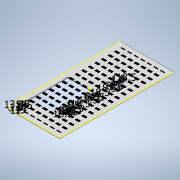
# Autodesk Inventor part: Backboard
Saved by Autodesk Inventor 2021 (Build 250183000, 183)
## iProperties
Created: 2020-06-05
Part Number: Backboard
Material: Generic
Document SubType Name: Modeling
Designer: ameli
Density: 1 g/cm^3
Appearance: Default
Author: ameli
Autodesk Inventor part; units mm, degrees
ref_plane "YZ Plane" through (0, 0, 0) normal (1, 0, 0) x (0, 1, 0)
ref_plane "XZ Plane" through (0, 0, 0) normal (0, 1, 0) x (-1, 0, 0)
ref_plane "XY Plane" through (0, 0, 0) normal (0, 0, 1) x (1, 0, 0)
sketch "Sketch1" plane through (0, 0, 0) normal (0, 1, 0) x (-1, 0, 0)
  line L0 (62, 129.5) -> (-60.5, 129.5)
  line L1 (-60.5, 129.5) -> (-60.5, -131.5)
  line L2 (-60.5, -131.5) -> (62, -131.5)
  line L3 (62, -131.5) -> (62, 129.5)
  point P0 (0, 0)
  dimension "d0" = 122.5
  dimension "d1" = 261
  dimension "d2" = 62
  dimension "d3" = 129.5
  constraints: 8 end point, 2 parallel, 1 horizontal, 1 perpendicular
  measures "d0" distance of L0.start L0.end
  measures "d1" distance of L2.end L0.start
  measures "d2" distance from line of point (0, 0) L3
  measures "d3" distance from line of point (0, 0) L0
extrude "Extrusion1" add sketch "Sketch1" along normal blind 2
sketch "Sketch6" plane through (0, 2, 0) normal (0, 1, 0) x (1, 0, 0)
  line L0 (-51, -88.5) -> (6, -88.5)
  line L1 (6, -88.5) -> (6, 0.5)
  line L2 (6, 0.5) -> (-51, 0.5)
  line L3 (-51, 0.5) -> (-51, -88.5)
  line L4 (-62, 131.5) -> (-62, -129.5) projected
  line L5 (-62, -129.5) -> (60.5, -129.5) projected
  point P0 (0, 0)
  dimension "d22" = 89
  dimension "d23" = 57
  dimension "d24" = 11
  dimension "d25" = 41
  constraints: 8 end point, 2 parallel, 1 horizontal, 1 perpendicular
  measures "d22" distance of L2.end L0.start
  measures "d23" distance of L0.start L0.end
  measures "d24" distance between parallel lines of L4 L3
  measures "d25" distance between parallel lines of L5 L0
extrude "Extrusion2" cut sketch "Sketch6" against normal blind 10
sketch "Sketch10" plane through (0, 2, 0) normal (0, 1, 0) x (1, 0, 0)
  line L0 (-48.25, -118.5) -> (-39.75, -118.5)
  line L1 (-39.75, -118.5) -> (-39.75, -117)
  line L2 (-39.75, -117) -> (-48.25, -117)
  line L3 (-48.25, -117) -> (-48.25, -118.5)
  line L4 (-48.25, -106) -> (-39.75, -106)
  line L5 (-39.75, -106) -> (-39.75, -104.5)
  line L6 (-39.75, -104.5) -> (-48.25, -104.5)
  line L7 (-48.25, -104.5) -> (-48.25, -106)
  line L8 (-62, 131.5) -> (-62, -129.5) projected
  line L9 (-62, -129.5) -> (60.5, -129.5) projected
  line L10 (-48.25, -103.5) -> (-39.75, -103.5)
  line L11 (-39.75, -103.5) -> (-39.75, -102)
  line L12 (-39.75, -102) -> (-48.25, -102)
  line L13 (-48.25, -102) -> (-48.25, -103.5)
  line L14 (-48.25, -91) -> (-39.75, -91)
  line L15 (-39.75, -91) -> (-39.75, -89.5)
  line L16 (-39.75, -89.5) -> (-48.25, -89.5)
  line L17 (-48.25, -89.5) -> (-48.25, -91)
  line L18 (-48.25, -88.5) -> (-39.75, -88.5)
  line L19 (-39.75, -88.5) -> (-39.75, -87)
  line L20 (-39.75, -87) -> (-48.25, -87)
  line L21 (-48.25, -87) -> (-48.25, -88.5)
  line L22 (-48.25, -76) -> (-39.75, -76)
  line L23 (-39.75, -76) -> (-39.75, -74.5)
  line L24 (-39.75, -74.5) -> (-48.25, -74.5)
  line L25 (-48.25, -74.5) -> (-48.25, -76)
  line L26 (-48.25, -73.5) -> (-39.75, -73.5)
  line L27 (-39.75, -73.5) -> (-39.75, -72)
  line L28 (-39.75, -72) -> (-48.25, -72)
  line L29 (-48.25, -72) -> (-48.25, -73.5)
  line L30 (-48.25, -61) -> (-39.75, -61)
  line L31 (-39.75, -61) -> (-39.75, -59.5)
  line L32 (-39.75, -59.5) -> (-48.25, -59.5)
  line L33 (-48.25, -59.5) -> (-48.25, -61)
  line L34 (-48.25, -58.5) -> (-39.75, -58.5)
  line L35 (-39.75, -58.5) -> (-39.75, -57)
  line L36 (-39.75, -57) -> (-48.25, -57)
  line L37 (-48.25, -57) -> (-48.25, -58.5)
  line L38 (-48.25, -46) -> (-39.75, -46)
  line L39 (-39.75, -46) -> (-39.75, -44.5)
  line L40 (-39.75, -44.5) -> (-48.25, -44.5)
  line L41 (-48.25, -44.5) -> (-48.25, -46)
  line L42 (-48.25, -43.5) -> (-39.75, -43.5)
  line L43 (-39.75, -43.5) -> (-39.75, -42)
  line L44 (-39.75, -42) -> (-48.25, -42)
  line L45 (-48.25, -42) -> (-48.25, -43.5)
  line L46 (-48.25, -31) -> (-39.75, -31)
  line L47 (-39.75, -31) -> (-39.75, -29.5)
  line L48 (-39.75, -29.5) -> (-48.25, -29.5)
  line L49 (-48.25, -29.5) -> (-48.25, -31)
  line L50 (-48.25, -28.5) -> (-39.75, -28.5)
  line L51 (-39.75, -28.5) -> (-39.75, -27)
  line L52 (-39.75, -27) -> (-48.25, -27)
  line L53 (-48.25, -27) -> (-48.25, -28.5)
  line L54 (-48.25, -16) -> (-39.75, -16)
  line L55 (-39.75, -16) -> (-39.75, -14.5)
  line L56 (-39.75, -14.5) -> (-48.25, -14.5)
  line L57 (-48.25, -14.5) -> (-48.25, -16)
  line L58 (-48.25, -13.5) -> (-39.75, -13.5)
  line L59 (-39.75, -13.5) -> (-39.75, -12)
  line L60 (-39.75, -12) -> (-48.25, -12)
  line L61 (-48.25, -12) -> (-48.25, -13.5)
  line L62 (-48.25, -1) -> (-39.75, -1)
  line L63 (-39.75, -1) -> (-39.75, 0.5)
  line L64 (-39.75, 0.5) -> (-48.25, 0.5)
  line L65 (-48.25, 0.5) -> (-48.25, -1)
  line L66 (-48.25, 1.5) -> (-39.75, 1.5)
  line L67 (-39.75, 1.5) -> (-39.75, 3)
  line L68 (-39.75, 3) -> (-48.25, 3)
  line L69 (-48.25, 3) -> (-48.25, 1.5)
  line L70 (-48.25, 14) -> (-39.75, 14)
  line L71 (-39.75, 14) -> (-39.75, 15.5)
  line L72 (-39.75, 15.5) -> (-48.25, 15.5)
  line L73 (-48.25, 15.5) -> (-48.25, 14)
  line L74 (-48.25, 16.5) -> (-39.75, 16.5)
  line L75 (-39.75, 16.5) -> (-39.75, 18)
  line L76 (-39.75, 18) -> (-48.25, 18)
  line L77 (-48.25, 18) -> (-48.25, 16.5)
  line L78 (-48.25, 29) -> (-39.75, 29)
  line L79 (-39.75, 29) -> (-39.75, 30.5)
  line L80 (-39.75, 30.5) -> (-48.25, 30.5)
  line L81 (-48.25, 30.5) -> (-48.25, 29)
  line L82 (-48.25, 31.5) -> (-39.75, 31.5)
  line L83 (-39.75, 31.5) -> (-39.75, 33)
  line L84 (-39.75, 33) -> (-48.25, 33)
  line L85 (-48.25, 33) -> (-48.25, 31.5)
  line L86 (-48.25, 44) -> (-39.75, 44)
  line L87 (-39.75, 44) -> (-39.75, 45.5)
  line L88 (-39.75, 45.5) -> (-48.25, 45.5)
  line L89 (-48.25, 45.5) -> (-48.25, 44)
  line L90 (-48.25, 46.5) -> (-39.75, 46.5)
  line L91 (-39.75, 46.5) -> (-39.75, 48)
  line L92 (-39.75, 48) -> (-48.25, 48)
  line L93 (-48.25, 48) -> (-48.25, 46.5)
  line L94 (-48.25, 59) -> (-39.75, 59)
  line L95 (-39.75, 59) -> (-39.75, 60.5)
  line L96 (-39.75, 60.5) -> (-48.25, 60.5)
  line L97 (-48.25, 60.5) -> (-48.25, 59)
  line L98 (-48.25, 61.5) -> (-39.75, 61.5)
  line L99 (-39.75, 61.5) -> (-39.75, 63)
  line L100 (-39.75, 63) -> (-48.25, 63)
  line L101 (-48.25, 63) -> (-48.25, 61.5)
  line L102 (-48.25, 74) -> (-39.75, 74)
  line L103 (-39.75, 74) -> (-39.75, 75.5)
  line L104 (-39.75, 75.5) -> (-48.25, 75.5)
  line L105 (-48.25, 75.5) -> (-48.25, 74)
  line L106 (-48.25, 76.5) -> (-39.75, 76.5)
  line L107 (-39.75, 76.5) -> (-39.75, 78)
  line L108 (-39.75, 78) -> (-48.25, 78)
  line L109 (-48.25, 78) -> (-48.25, 76.5)
  line L110 (-48.25, 89) -> (-39.75, 89)
  line L111 (-39.75, 89) -> (-39.75, 90.5)
  line L112 (-39.75, 90.5) -> (-48.25, 90.5)
  line L113 (-48.25, 90.5) -> (-48.25, 89)
  line L114 (-48.25, 91.5) -> (-39.75, 91.5)
  line L115 (-39.75, 91.5) -> (-39.75, 93)
  line L116 (-39.75, 93) -> (-48.25, 93)
  line L117 (-48.25, 93) -> (-48.25, 91.5)
  line L118 (-48.25, 104) -> (-39.75, 104)
  line L119 (-39.75, 104) -> (-39.75, 105.5)
  line L120 (-39.75, 105.5) -> (-48.25, 105.5)
  line L121 (-48.25, 105.5) -> (-48.25, 104)
  line L122 (-48.25, 106.5) -> (-39.75, 106.5)
  line L123 (-39.75, 106.5) -> (-39.75, 108)
  line L124 (-39.75, 108) -> (-48.25, 108)
  line L125 (-48.25, 108) -> (-48.25, 106.5)
  line L126 (-48.25, 119) -> (-39.75, 119)
  line L127 (-39.75, 119) -> (-39.75, 120.5)
  line L128 (-39.75, 120.5) -> (-48.25, 120.5)
  line L129 (-48.25, 120.5) -> (-48.25, 119)
  line L130 (-33.25, -118.5) -> (-24.75, -118.5)
  line L131 (-24.75, -118.5) -> (-24.75, -117)
  line L132 (-24.75, -117) -> (-33.25, -117)
  line L133 (-33.25, -117) -> (-33.25, -118.5)
  line L134 (-33.25, -106) -> (-24.75, -106)
  line L135 (-24.75, -106) -> (-24.75, -104.5)
  line L136 (-24.75, -104.5) -> (-33.25, -104.5)
  line L137 (-33.25, -104.5) -> (-33.25, -106)
  line L138 (-33.25, -103.5) -> (-24.75, -103.5)
  line L139 (-24.75, -103.5) -> (-24.75, -102)
  line L140 (-24.75, -102) -> (-33.25, -102)
  line L141 (-33.25, -102) -> (-33.25, -103.5)
  line L142 (-33.25, -91) -> (-24.75, -91)
  line L143 (-24.75, -91) -> (-24.75, -89.5)
  line L144 (-24.75, -89.5) -> (-33.25, -89.5)
  line L145 (-33.25, -89.5) -> (-33.25, -91)
  line L146 (-33.25, -88.5) -> (-24.75, -88.5)
  line L147 (-24.75, -88.5) -> (-24.75, -87)
  line L148 (-24.75, -87) -> (-33.25, -87)
  line L149 (-33.25, -87) -> (-33.25, -88.5)
  line L150 (-33.25, -76) -> (-24.75, -76)
  line L151 (-24.75, -76) -> (-24.75, -74.5)
  line L152 (-24.75, -74.5) -> (-33.25, -74.5)
  line L153 (-33.25, -74.5) -> (-33.25, -76)
  line L154 (-33.25, -73.5) -> (-24.75, -73.5)
  line L155 (-24.75, -73.5) -> (-24.75, -72)
  line L156 (-24.75, -72) -> (-33.25, -72)
  line L157 (-33.25, -72) -> (-33.25, -73.5)
  line L158 (-33.25, -61) -> (-24.75, -61)
  line L159 (-24.75, -61) -> (-24.75, -59.5)
  line L160 (-24.75, -59.5) -> (-33.25, -59.5)
  line L161 (-33.25, -59.5) -> (-33.25, -61)
  line L162 (-33.25, -58.5) -> (-24.75, -58.5)
  line L163 (-24.75, -58.5) -> (-24.75, -57)
  line L164 (-24.75, -57) -> (-33.25, -57)
  line L165 (-33.25, -57) -> (-33.25, -58.5)
  line L166 (-33.25, -46) -> (-24.75, -46)
  line L167 (-24.75, -46) -> (-24.75, -44.5)
  line L168 (-24.75, -44.5) -> (-33.25, -44.5)
  line L169 (-33.25, -44.5) -> (-33.25, -46)
  line L170 (-33.25, -43.5) -> (-24.75, -43.5)
  line L171 (-24.75, -43.5) -> (-24.75, -42)
  line L172 (-24.75, -42) -> (-33.25, -42)
  line L173 (-33.25, -42) -> (-33.25, -43.5)
  line L174 (-33.25, -31) -> (-24.75, -31)
  line L175 (-24.75, -31) -> (-24.75, -29.5)
  line L176 (-24.75, -29.5) -> (-33.25, -29.5)
  line L177 (-33.25, -29.5) -> (-33.25, -31)
  line L178 (-33.25, -28.5) -> (-24.75, -28.5)
  line L179 (-24.75, -28.5) -> (-24.75, -27)
  line L180 (-24.75, -27) -> (-33.25, -27)
  line L181 (-33.25, -27) -> (-33.25, -28.5)
  line L182 (-33.25, -16) -> (-24.75, -16)
  line L183 (-24.75, -16) -> (-24.75, -14.5)
  line L184 (-24.75, -14.5) -> (-33.25, -14.5)
  line L185 (-33.25, -14.5) -> (-33.25, -16)
  line L186 (-33.25, -13.5) -> (-24.75, -13.5)
  line L187 (-24.75, -13.5) -> (-24.75, -12)
  line L188 (-24.75, -12) -> (-33.25, -12)
  line L189 (-33.25, -12) -> (-33.25, -13.5)
  line L190 (-33.25, -1) -> (-24.75, -1)
  line L191 (-24.75, -1) -> (-24.75, 0.5)
  line L192 (-24.75, 0.5) -> (-33.25, 0.5)
  line L193 (-33.25, 0.5) -> (-33.25, -1)
  line L194 (-33.25, 1.5) -> (-24.75, 1.5)
  line L195 (-24.75, 1.5) -> (-24.75, 3)
  line L196 (-24.75, 3) -> (-33.25, 3)
  line L197 (-33.25, 3) -> (-33.25, 1.5)
  line L198 (-33.25, 14) -> (-24.75, 14)
  line L199 (-24.75, 14) -> (-24.75, 15.5)
  line L200 (-24.75, 15.5) -> (-33.25, 15.5)
  line L201 (-33.25, 15.5) -> (-33.25, 14)
  line L202 (-33.25, 16.5) -> (-24.75, 16.5)
  line L203 (-24.75, 16.5) -> (-24.75, 18)
  line L204 (-24.75, 18) -> (-33.25, 18)
  line L205 (-33.25, 18) -> (-33.25, 16.5)
  line L206 (-33.25, 29) -> (-24.75, 29)
  line L207 (-24.75, 29) -> (-24.75, 30.5)
  line L208 (-24.75, 30.5) -> (-33.25, 30.5)
  line L209 (-33.25, 30.5) -> (-33.25, 29)
  line L210 (-33.25, 31.5) -> (-24.75, 31.5)
  line L211 (-24.75, 31.5) -> (-24.75, 33)
  line L212 (-24.75, 33) -> (-33.25, 33)
  line L213 (-33.25, 33) -> (-33.25, 31.5)
  line L214 (-33.25, 44) -> (-24.75, 44)
  line L215 (-24.75, 44) -> (-24.75, 45.5)
  line L216 (-24.75, 45.5) -> (-33.25, 45.5)
  line L217 (-33.25, 45.5) -> (-33.25, 44)
  line L218 (-33.25, 46.5) -> (-24.75, 46.5)
  line L219 (-24.75, 46.5) -> (-24.75, 48)
  line L220 (-24.75, 48) -> (-33.25, 48)
  line L221 (-33.25, 48) -> (-33.25, 46.5)
  line L222 (-33.25, 59) -> (-24.75, 59)
  line L223 (-24.75, 59) -> (-24.75, 60.5)
  line L224 (-24.75, 60.5) -> (-33.25, 60.5)
  line L225 (-33.25, 60.5) -> (-33.25, 59)
  line L226 (-33.25, 61.5) -> (-24.75, 61.5)
  line L227 (-24.75, 61.5) -> (-24.75, 63)
  line L228 (-24.75, 63) -> (-33.25, 63)
  line L229 (-33.25, 63) -> (-33.25, 61.5)
  line L230 (-33.25, 74) -> (-24.75, 74)
  line L231 (-24.75, 74) -> (-24.75, 75.5)
  line L232 (-24.75, 75.5) -> (-33.25, 75.5)
  line L233 (-33.25, 75.5) -> (-33.25, 74)
  line L234 (-33.25, 76.5) -> (-24.75, 76.5)
  line L235 (-24.75, 76.5) -> (-24.75, 78)
  line L236 (-24.75, 78) -> (-33.25, 78)
  line L237 (-33.25, 78) -> (-33.25, 76.5)
  line L238 (-33.25, 89) -> (-24.75, 89)
  line L239 (-24.75, 89) -> (-24.75, 90.5)
  line L240 (-24.75, 90.5) -> (-33.25, 90.5)
  line L241 (-33.25, 90.5) -> (-33.25, 89)
  line L242 (-33.25, 91.5) -> (-24.75, 91.5)
  line L243 (-24.75, 91.5) -> (-24.75, 93)
  line L244 (-24.75, 93) -> (-33.25, 93)
  line L245 (-33.25, 93) -> (-33.25, 91.5)
  line L246 (-33.25, 104) -> (-24.75, 104)
  line L247 (-24.75, 104) -> (-24.75, 105.5)
  line L248 (-24.75, 105.5) -> (-33.25, 105.5)
  line L249 (-33.25, 105.5) -> (-33.25, 104)
  line L250 (-33.25, 106.5) -> (-24.75, 106.5)
  line L251 (-24.75, 106.5) -> (-24.75, 108)
  line L252 (-24.75, 108) -> (-33.25, 108)
  line L253 (-33.25, 108) -> (-33.25, 106.5)
  line L254 (-33.25, 119) -> (-24.75, 119)
  line L255 (-24.75, 119) -> (-24.75, 120.5)
  line L256 (-24.75, 120.5) -> (-33.25, 120.5)
  line L257 (-33.25, 120.5) -> (-33.25, 119)
  line L258 (-18.25, -118.5) -> (-9.75, -118.5)
  line L259 (-9.75, -118.5) -> (-9.75, -117)
  line L260 (-9.75, -117) -> (-18.25, -117)
  line L261 (-18.25, -117) -> (-18.25, -118.5)
  line L262 (-18.25, -106) -> (-9.75, -106)
  line L263 (-9.75, -106) -> (-9.75, -104.5)
  line L264 (-9.75, -104.5) -> (-18.25, -104.5)
  line L265 (-18.25, -104.5) -> (-18.25, -106)
  line L266 (-18.25, -103.5) -> (-9.75, -103.5)
  line L267 (-9.75, -103.5) -> (-9.75, -102)
  line L268 (-9.75, -102) -> (-18.25, -102)
  line L269 (-18.25, -102) -> (-18.25, -103.5)
  line L270 (-18.25, -91) -> (-9.75, -91)
  line L271 (-9.75, -91) -> (-9.75, -89.5)
  line L272 (-9.75, -89.5) -> (-18.25, -89.5)
  line L273 (-18.25, -89.5) -> (-18.25, -91)
  line L274 (-18.25, -88.5) -> (-9.75, -88.5)
  line L275 (-9.75, -88.5) -> (-9.75, -87)
  line L276 (-9.75, -87) -> (-18.25, -87)
  line L277 (-18.25, -87) -> (-18.25, -88.5)
  line L278 (-18.25, -76) -> (-9.75, -76)
  line L279 (-9.75, -76) -> (-9.75, -74.5)
  line L280 (-9.75, -74.5) -> (-18.25, -74.5)
  line L281 (-18.25, -74.5) -> (-18.25, -76)
  line L282 (-18.25, -73.5) -> (-9.75, -73.5)
  line L283 (-9.75, -73.5) -> (-9.75, -72)
  line L284 (-9.75, -72) -> (-18.25, -72)
  line L285 (-18.25, -72) -> (-18.25, -73.5)
  line L286 (-18.25, -61) -> (-9.75, -61)
  line L287 (-9.75, -61) -> (-9.75, -59.5)
  line L288 (-9.75, -59.5) -> (-18.25, -59.5)
  line L289 (-18.25, -59.5) -> (-18.25, -61)
  line L290 (-18.25, -58.5) -> (-9.75, -58.5)
  line L291 (-9.75, -58.5) -> (-9.75, -57)
  line L292 (-9.75, -57) -> (-18.25, -57)
  line L293 (-18.25, -57) -> (-18.25, -58.5)
  line L294 (-18.25, -46) -> (-9.75, -46)
  line L295 (-9.75, -46) -> (-9.75, -44.5)
  line L296 (-9.75, -44.5) -> (-18.25, -44.5)
  line L297 (-18.25, -44.5) -> (-18.25, -46)
  line L298 (-18.25, -43.5) -> (-9.75, -43.5)
  line L299 (-9.75, -43.5) -> (-9.75, -42)
  line L300 (-9.75, -42) -> (-18.25, -42)
  line L301 (-18.25, -42) -> (-18.25, -43.5)
  line L302 (-18.25, -31) -> (-9.75, -31)
  line L303 (-9.75, -31) -> (-9.75, -29.5)
  line L304 (-9.75, -29.5) -> (-18.25, -29.5)
  line L305 (-18.25, -29.5) -> (-18.25, -31)
  line L306 (-18.25, -28.5) -> (-9.75, -28.5)
  line L307 (-9.75, -28.5) -> (-9.75, -27)
  line L308 (-9.75, -27) -> (-18.25, -27)
  line L309 (-18.25, -27) -> (-18.25, -28.5)
  line L310 (-18.25, -16) -> (-9.75, -16)
  line L311 (-9.75, -16) -> (-9.75, -14.5)
  line L312 (-9.75, -14.5) -> (-18.25, -14.5)
  line L313 (-18.25, -14.5) -> (-18.25, -16)
  line L314 (-18.25, -13.5) -> (-9.75, -13.5)
  line L315 (-9.75, -13.5) -> (-9.75, -12)
  line L316 (-9.75, -12) -> (-18.25, -12)
  line L317 (-18.25, -12) -> (-18.25, -13.5)
  line L318 (-18.25, -1) -> (-9.75, -1)
  line L319 (-9.75, -1) -> (-9.75, 0.5)
  line L320 (-9.75, 0.5) -> (-18.25, 0.5)
  line L321 (-18.25, 0.5) -> (-18.25, -1)
  line L322 (-18.25, 1.5) -> (-9.75, 1.5)
  line L323 (-9.75, 1.5) -> (-9.75, 3)
  line L324 (-9.75, 3) -> (-18.25, 3)
  line L325 (-18.25, 3) -> (-18.25, 1.5)
  line L326 (-18.25, 14) -> (-9.75, 14)
  line L327 (-9.75, 14) -> (-9.75, 15.5)
  line L328 (-9.75, 15.5) -> (-18.25, 15.5)
  line L329 (-18.25, 15.5) -> (-18.25, 14)
  line L330 (-18.25, 16.5) -> (-9.75, 16.5)
  line L331 (-9.75, 16.5) -> (-9.75, 18)
  line L332 (-9.75, 18) -> (-18.25, 18)
  line L333 (-18.25, 18) -> (-18.25, 16.5)
  line L334 (-18.25, 29) -> (-9.75, 29)
  line L335 (-9.75, 29) -> (-9.75, 30.5)
  line L336 (-9.75, 30.5) -> (-18.25, 30.5)
  line L337 (-18.25, 30.5) -> (-18.25, 29)
  line L338 (-18.25, 31.5) -> (-9.75, 31.5)
  line L339 (-9.75, 31.5) -> (-9.75, 33)
  line L340 (-9.75, 33) -> (-18.25, 33)
  line L341 (-18.25, 33) -> (-18.25, 31.5)
  line L342 (-18.25, 44) -> (-9.75, 44)
  line L343 (-9.75, 44) -> (-9.75, 45.5)
  line L344 (-9.75, 45.5) -> (-18.25, 45.5)
  line L345 (-18.25, 45.5) -> (-18.25, 44)
  line L346 (-18.25, 46.5) -> (-9.75, 46.5)
  line L347 (-9.75, 46.5) -> (-9.75, 48)
  line L348 (-9.75, 48) -> (-18.25, 48)
  line L349 (-18.25, 48) -> (-18.25, 46.5)
  line L350 (-18.25, 59) -> (-9.75, 59)
  line L351 (-9.75, 59) -> (-9.75, 60.5)
  line L352 (-9.75, 60.5) -> (-18.25, 60.5)
  line L353 (-18.25, 60.5) -> (-18.25, 59)
  line L354 (-18.25, 61.5) -> (-9.75, 61.5)
  line L355 (-9.75, 61.5) -> (-9.75, 63)
  line L356 (-9.75, 63) -> (-18.25, 63)
  line L357 (-18.25, 63) -> (-18.25, 61.5)
  line L358 (-18.25, 74) -> (-9.75, 74)
  line L359 (-9.75, 74) -> (-9.75, 75.5)
  line L360 (-9.75, 75.5) -> (-18.25, 75.5)
  line L361 (-18.25, 75.5) -> (-18.25, 74)
  line L362 (-18.25, 76.5) -> (-9.75, 76.5)
  line L363 (-9.75, 76.5) -> (-9.75, 78)
  line L364 (-9.75, 78) -> (-18.25, 78)
  line L365 (-18.25, 78) -> (-18.25, 76.5)
  line L366 (-18.25, 89) -> (-9.75, 89)
  line L367 (-9.75, 89) -> (-9.75, 90.5)
  line L368 (-9.75, 90.5) -> (-18.25, 90.5)
  line L369 (-18.25, 90.5) -> (-18.25, 89)
  line L370 (-18.25, 91.5) -> (-9.75, 91.5)
  line L371 (-9.75, 91.5) -> (-9.75, 93)
  line L372 (-9.75, 93) -> (-18.25, 93)
  line L373 (-18.25, 93) -> (-18.25, 91.5)
  line L374 (-18.25, 104) -> (-9.75, 104)
  line L375 (-9.75, 104) -> (-9.75, 105.5)
  line L376 (-9.75, 105.5) -> (-18.25, 105.5)
  line L377 (-18.25, 105.5) -> (-18.25, 104)
  line L378 (-18.25, 106.5) -> (-9.75, 106.5)
  line L379 (-9.75, 106.5) -> (-9.75, 108)
  line L380 (-9.75, 108) -> (-18.25, 108)
  line L381 (-18.25, 108) -> (-18.25, 106.5)
  line L382 (-18.25, 119) -> (-9.75, 119)
  line L383 (-9.75, 119) -> (-9.75, 120.5)
  line L384 (-9.75, 120.5) -> (-18.25, 120.5)
  line L385 (-18.25, 120.5) -> (-18.25, 119)
  line L386 (-3.25, -118.5) -> (5.25, -118.5)
  line L387 (5.25, -118.5) -> (5.25, -117)
  line L388 (5.25, -117) -> (-3.25, -117)
  line L389 (-3.25, -117) -> (-3.25, -118.5)
  line L390 (-3.25, -106) -> (5.25, -106)
  line L391 (5.25, -106) -> (5.25, -104.5)
  line L392 (5.25, -104.5) -> (-3.25, -104.5)
  line L393 (-3.25, -104.5) -> (-3.25, -106)
  line L394 (-3.25, -103.5) -> (5.25, -103.5)
  line L395 (5.25, -103.5) -> (5.25, -102)
  line L396 (5.25, -102) -> (-3.25, -102)
  line L397 (-3.25, -102) -> (-3.25, -103.5)
  line L398 (-3.25, -91) -> (5.25, -91)
  line L399 (5.25, -91) -> (5.25, -89.5)
  line L400 (5.25, -89.5) -> (-3.25, -89.5)
  line L401 (-3.25, -89.5) -> (-3.25, -91)
  line L402 (-3.25, -88.5) -> (5.25, -88.5)
  line L403 (5.25, -88.5) -> (5.25, -87)
  line L404 (5.25, -87) -> (-3.25, -87)
  line L405 (-3.25, -87) -> (-3.25, -88.5)
  line L406 (-3.25, -76) -> (5.25, -76)
  line L407 (5.25, -76) -> (5.25, -74.5)
  line L408 (5.25, -74.5) -> (-3.25, -74.5)
  line L409 (-3.25, -74.5) -> (-3.25, -76)
  line L410 (-3.25, -73.5) -> (5.25, -73.5)
  line L411 (5.25, -73.5) -> (5.25, -72)
  line L412 (5.25, -72) -> (-3.25, -72)
  line L413 (-3.25, -72) -> (-3.25, -73.5)
  line L414 (-3.25, -61) -> (5.25, -61)
  line L415 (5.25, -61) -> (5.25, -59.5)
  line L416 (5.25, -59.5) -> (-3.25, -59.5)
  line L417 (-3.25, -59.5) -> (-3.25, -61)
  line L418 (-3.25, -58.5) -> (5.25, -58.5)
  line L419 (5.25, -58.5) -> (5.25, -57)
  line L420 (5.25, -57) -> (-3.25, -57)
  line L421 (-3.25, -57) -> (-3.25, -58.5)
  line L422 (-3.25, -46) -> (5.25, -46)
  line L423 (5.25, -46) -> (5.25, -44.5)
  line L424 (5.25, -44.5) -> (-3.25, -44.5)
  line L425 (-3.25, -44.5) -> (-3.25, -46)
  line L426 (-3.25, -43.5) -> (5.25, -43.5)
  line L427 (5.25, -43.5) -> (5.25, -42)
  line L428 (5.25, -42) -> (-3.25, -42)
  line L429 (-3.25, -42) -> (-3.25, -43.5)
  line L430 (-3.25, -31) -> (5.25, -31)
  line L431 (5.25, -31) -> (5.25, -29.5)
  line L432 (5.25, -29.5) -> (-3.25, -29.5)
  line L433 (-3.25, -29.5) -> (-3.25, -31)
  line L434 (-3.25, -28.5) -> (5.25, -28.5)
  line L435 (5.25, -28.5) -> (5.25, -27)
  line L436 (5.25, -27) -> (-3.25, -27)
  line L437 (-3.25, -27) -> (-3.25, -28.5)
  line L438 (-3.25, -16) -> (5.25, -16)
  line L439 (5.25, -16) -> (5.25, -14.5)
  line L440 (5.25, -14.5) -> (-3.25, -14.5)
  line L441 (-3.25, -14.5) -> (-3.25, -16)
  line L442 (-3.25, -13.5) -> (5.25, -13.5)
  line L443 (5.25, -13.5) -> (5.25, -12)
  line L444 (5.25, -12) -> (-3.25, -12)
  line L445 (-3.25, -12) -> (-3.25, -13.5)
  line L446 (-3.25, -1) -> (5.25, -1)
  line L447 (5.25, -1) -> (5.25, 0.5)
  line L448 (5.25, 0.5) -> (-3.25, 0.5)
  line L449 (-3.25, 0.5) -> (-3.25, -1)
  line L450 (-3.25, 1.5) -> (5.25, 1.5)
  line L451 (5.25, 1.5) -> (5.25, 3)
  line L452 (5.25, 3) -> (-3.25, 3)
  line L453 (-3.25, 3) -> (-3.25, 1.5)
  line L454 (-3.25, 14) -> (5.25, 14)
  line L455 (5.25, 14) -> (5.25, 15.5)
  line L456 (5.25, 15.5) -> (-3.25, 15.5)
  line L457 (-3.25, 15.5) -> (-3.25, 14)
  line L458 (-3.25, 16.5) -> (5.25, 16.5)
  line L459 (5.25, 16.5) -> (5.25, 18)
  line L460 (5.25, 18) -> (-3.25, 18)
  line L461 (-3.25, 18) -> (-3.25, 16.5)
  line L462 (-3.25, 29) -> (5.25, 29)
  line L463 (5.25, 29) -> (5.25, 30.5)
  line L464 (5.25, 30.5) -> (-3.25, 30.5)
  line L465 (-3.25, 30.5) -> (-3.25, 29)
  line L466 (-3.25, 31.5) -> (5.25, 31.5)
  line L467 (5.25, 31.5) -> (5.25, 33)
  line L468 (5.25, 33) -> (-3.25, 33)
  line L469 (-3.25, 33) -> (-3.25, 31.5)
  line L470 (-3.25, 44) -> (5.25, 44)
  line L471 (5.25, 44) -> (5.25, 45.5)
  line L472 (5.25, 45.5) -> (-3.25, 45.5)
  line L473 (-3.25, 45.5) -> (-3.25, 44)
  line L474 (-3.25, 46.5) -> (5.25, 46.5)
  line L475 (5.25, 46.5) -> (5.25, 48)
  line L476 (5.25, 48) -> (-3.25, 48)
  line L477 (-3.25, 48) -> (-3.25, 46.5)
  line L478 (-3.25, 59) -> (5.25, 59)
  line L479 (5.25, 59) -> (5.25, 60.5)
  line L480 (5.25, 60.5) -> (-3.25, 60.5)
  line L481 (-3.25, 60.5) -> (-3.25, 59)
  line L482 (-3.25, 61.5) -> (5.25, 61.5)
  line L483 (5.25, 61.5) -> (5.25, 63)
  line L484 (5.25, 63) -> (-3.25, 63)
  line L485 (-3.25, 63) -> (-3.25, 61.5)
  line L486 (-3.25, 74) -> (5.25, 74)
  line L487 (5.25, 74) -> (5.25, 75.5)
  line L488 (5.25, 75.5) -> (-3.25, 75.5)
  line L489 (-3.25, 75.5) -> (-3.25, 74)
  line L490 (-3.25, 76.5) -> (5.25, 76.5)
  line L491 (5.25, 76.5) -> (5.25, 78)
  line L492 (5.25, 78) -> (-3.25, 78)
  line L493 (-3.25, 78) -> (-3.25, 76.5)
  line L494 (-3.25, 89) -> (5.25, 89)
  line L495 (5.25, 89) -> (5.25, 90.5)
  line L496 (5.25, 90.5) -> (-3.25, 90.5)
  line L497 (-3.25, 90.5) -> (-3.25, 89)
  line L498 (-3.25, 91.5) -> (5.25, 91.5)
  line L499 (5.25, 91.5) -> (5.25, 93)
  line L500 (5.25, 93) -> (-3.25, 93)
  line L501 (-3.25, 93) -> (-3.25, 91.5)
  line L502 (-3.25, 104) -> (5.25, 104)
  line L503 (5.25, 104) -> (5.25, 105.5)
  line L504 (5.25, 105.5) -> (-3.25, 105.5)
  line L505 (-3.25, 105.5) -> (-3.25, 104)
  line L506 (-3.25, 106.5) -> (5.25, 106.5)
  line L507 (5.25, 106.5) -> (5.25, 108)
  line L508 (5.25, 108) -> (-3.25, 108)
  line L509 (-3.25, 108) -> (-3.25, 106.5)
  line L510 (-3.25, 119) -> (5.25, 119)
  line L511 (5.25, 119) -> (5.25, 120.5)
  line L512 (5.25, 120.5) -> (-3.25, 120.5)
  line L513 (-3.25, 120.5) -> (-3.25, 119)
  line L514 (11.75, -118.5) -> (20.25, -118.5)
  line L515 (20.25, -118.5) -> (20.25, -117)
  line L516 (20.25, -117) -> (11.75, -117)
  line L517 (11.75, -117) -> (11.75, -118.5)
  line L518 (11.75, -106) -> (20.25, -106)
  line L519 (20.25, -106) -> (20.25, -104.5)
  line L520 (20.25, -104.5) -> (11.75, -104.5)
  line L521 (11.75, -104.5) -> (11.75, -106)
  line L522 (11.75, -103.5) -> (20.25, -103.5)
  line L523 (20.25, -103.5) -> (20.25, -102)
  line L524 (20.25, -102) -> (11.75, -102)
  line L525 (11.75, -102) -> (11.75, -103.5)
  line L526 (11.75, -91) -> (20.25, -91)
  line L527 (20.25, -91) -> (20.25, -89.5)
  line L528 (20.25, -89.5) -> (11.75, -89.5)
  line L529 (11.75, -89.5) -> (11.75, -91)
  line L530 (11.75, -88.5) -> (20.25, -88.5)
  line L531 (20.25, -88.5) -> (20.25, -87)
  line L532 (20.25, -87) -> (11.75, -87)
  line L533 (11.75, -87) -> (11.75, -88.5)
  line L534 (11.75, -76) -> (20.25, -76)
  line L535 (20.25, -76) -> (20.25, -74.5)
  line L536 (20.25, -74.5) -> (11.75, -74.5)
  line L537 (11.75, -74.5) -> (11.75, -76)
  line L538 (11.75, -73.5) -> (20.25, -73.5)
  line L539 (20.25, -73.5) -> (20.25, -72)
  line L540 (20.25, -72) -> (11.75, -72)
  line L541 (11.75, -72) -> (11.75, -73.5)
  line L542 (11.75, -61) -> (20.25, -61)
  line L543 (20.25, -61) -> (20.25, -59.5)
  line L544 (20.25, -59.5) -> (11.75, -59.5)
  line L545 (11.75, -59.5) -> (11.75, -61)
  line L546 (11.75, -58.5) -> (20.25, -58.5)
  line L547 (20.25, -58.5) -> (20.25, -57)
  line L548 (20.25, -57) -> (11.75, -57)
  line L549 (11.75, -57) -> (11.75, -58.5)
  line L550 (11.75, -46) -> (20.25, -46)
  line L551 (20.25, -46) -> (20.25, -44.5)
  line L552 (20.25, -44.5) -> (11.75, -44.5)
  line L553 (11.75, -44.5) -> (11.75, -46)
  line L554 (11.75, -43.5) -> (20.25, -43.5)
  line L555 (20.25, -43.5) -> (20.25, -42)
  line L556 (20.25, -42) -> (11.75, -42)
  line L557 (11.75, -42) -> (11.75, -43.5)
  line L558 (11.75, -31) -> (20.25, -31)
  line L559 (20.25, -31) -> (20.25, -29.5)
  line L560 (20.25, -29.5) -> (11.75, -29.5)
  line L561 (11.75, -29.5) -> (11.75, -31)
  line L562 (11.75, -28.5) -> (20.25, -28.5)
  line L563 (20.25, -28.5) -> (20.25, -27)
  line L564 (20.25, -27) -> (11.75, -27)
  line L565 (11.75, -27) -> (11.75, -28.5)
  line L566 (11.75, -16) -> (20.25, -16)
  line L567 (20.25, -16) -> (20.25, -14.5)
  line L568 (20.25, -14.5) -> (11.75, -14.5)
  line L569 (11.75, -14.5) -> (11.75, -16)
  line L570 (11.75, -13.5) -> (20.25, -13.5)
  line L571 (20.25, -13.5) -> (20.25, -12)
  line L572 (20.25, -12) -> (11.75, -12)
  line L573 (11.75, -12) -> (11.75, -13.5)
  line L574 (11.75, -1) -> (20.25, -1)
  line L575 (20.25, -1) -> (20.25, 0.5)
  line L576 (20.25, 0.5) -> (11.75, 0.5)
  line L577 (11.75, 0.5) -> (11.75, -1)
  line L578 (11.75, 1.5) -> (20.25, 1.5)
  line L579 (20.25, 1.5) -> (20.25, 3)
  line L580 (20.25, 3) -> (11.75, 3)
  line L581 (11.75, 3) -> (11.75, 1.5)
  line L582 (11.75, 14) -> (20.25, 14)
  line L583 (20.25, 14) -> (20.25, 15.5)
  line L584 (20.25, 15.5) -> (11.75, 15.5)
  line L585 (11.75, 15.5) -> (11.75, 14)
  line L586 (11.75, 16.5) -> (20.25, 16.5)
  line L587 (20.25, 16.5) -> (20.25, 18)
  line L588 (20.25, 18) -> (11.75, 18)
  line L589 (11.75, 18) -> (11.75, 16.5)
  line L590 (11.75, 29) -> (20.25, 29)
  line L591 (20.25, 29) -> (20.25, 30.5)
  line L592 (20.25, 30.5) -> (11.75, 30.5)
  line L593 (11.75, 30.5) -> (11.75, 29)
  line L594 (11.75, 31.5) -> (20.25, 31.5)
  line L595 (20.25, 31.5) -> (20.25, 33)
  line L596 (20.25, 33) -> (11.75, 33)
  line L597 (11.75, 33) -> (11.75, 31.5)
  line L598 (11.75, 44) -> (20.25, 44)
  line L599 (20.25, 44) -> (20.25, 45.5)
  line L600 (20.25, 45.5) -> (11.75, 45.5)
  line L601 (11.75, 45.5) -> (11.75, 44)
  line L602 (11.75, 46.5) -> (20.25, 46.5)
  line L603 (20.25, 46.5) -> (20.25, 48)
  line L604 (20.25, 48) -> (11.75, 48)
  line L605 (11.75, 48) -> (11.75, 46.5)
  line L606 (11.75, 59) -> (20.25, 59)
  line L607 (20.25, 59) -> (20.25, 60.5)
  line L608 (20.25, 60.5) -> (11.75, 60.5)
  line L609 (11.75, 60.5) -> (11.75, 59)
  line L610 (11.75, 61.5) -> (20.25, 61.5)
  line L611 (20.25, 61.5) -> (20.25, 63)
  line L612 (20.25, 63) -> (11.75, 63)
  line L613 (11.75, 63) -> (11.75, 61.5)
  line L614 (11.75, 74) -> (20.25, 74)
  line L615 (20.25, 74) -> (20.25, 75.5)
  line L616 (20.25, 75.5) -> (11.75, 75.5)
  line L617 (11.75, 75.5) -> (11.75, 74)
  line L618 (11.75, 76.5) -> (20.25, 76.5)
  line L619 (20.25, 76.5) -> (20.25, 78)
  line L620 (20.25, 78) -> (11.75, 78)
  line L621 (11.75, 78) -> (11.75, 76.5)
  line L622 (11.75, 89) -> (20.25, 89)
  line L623 (20.25, 89) -> (20.25, 90.5)
  line L624 (20.25, 90.5) -> (11.75, 90.5)
  line L625 (11.75, 90.5) -> (11.75, 89)
  line L626 (11.75, 91.5) -> (20.25, 91.5)
  line L627 (20.25, 91.5) -> (20.25, 93)
  line L628 (20.25, 93) -> (11.75, 93)
  line L629 (11.75, 93) -> (11.75, 91.5)
  line L630 (11.75, 104) -> (20.25, 104)
  line L631 (20.25, 104) -> (20.25, 105.5)
  line L632 (20.25, 105.5) -> (11.75, 105.5)
  line L633 (11.75, 105.5) -> (11.75, 104)
  line L634 (11.75, 106.5) -> (20.25, 106.5)
  line L635 (20.25, 106.5) -> (20.25, 108)
  line L636 (20.25, 108) -> (11.75, 108)
  line L637 (11.75, 108) -> (11.75, 106.5)
  line L638 (11.75, 119) -> (20.25, 119)
  line L639 (20.25, 119) -> (20.25, 120.5)
  line L640 (20.25, 120.5) -> (11.75, 120.5)
  line L641 (11.75, 120.5) -> (11.75, 119)
  line L642 (26.75, -118.5) -> (35.25, -118.5)
  line L643 (35.25, -118.5) -> (35.25, -117)
  line L644 (35.25, -117) -> (26.75, -117)
  line L645 (26.75, -117) -> (26.75, -118.5)
  line L646 (26.75, -106) -> (35.25, -106)
  line L647 (35.25, -106) -> (35.25, -104.5)
  line L648 (35.25, -104.5) -> (26.75, -104.5)
  line L649 (26.75, -104.5) -> (26.75, -106)
  line L650 (26.75, -103.5) -> (35.25, -103.5)
  line L651 (35.25, -103.5) -> (35.25, -102)
  line L652 (35.25, -102) -> (26.75, -102)
  line L653 (26.75, -102) -> (26.75, -103.5)
  line L654 (26.75, -91) -> (35.25, -91)
  line L655 (35.25, -91) -> (35.25, -89.5)
  line L656 (35.25, -89.5) -> (26.75, -89.5)
  line L657 (26.75, -89.5) -> (26.75, -91)
  line L658 (26.75, -88.5) -> (35.25, -88.5)
  line L659 (35.25, -88.5) -> (35.25, -87)
  line L660 (35.25, -87) -> (26.75, -87)
  line L661 (26.75, -87) -> (26.75, -88.5)
  line L662 (26.75, -76) -> (35.25, -76)
  line L663 (35.25, -76) -> (35.25, -74.5)
  line L664 (35.25, -74.5) -> (26.75, -74.5)
  line L665 (26.75, -74.5) -> (26.75, -76)
  line L666 (26.75, -73.5) -> (35.25, -73.5)
  line L667 (35.25, -73.5) -> (35.25, -72)
  line L668 (35.25, -72) -> (26.75, -72)
  line L669 (26.75, -72) -> (26.75, -73.5)
  line L670 (26.75, -61) -> (35.25, -61)
  line L671 (35.25, -61) -> (35.25, -59.5)
  line L672 (35.25, -59.5) -> (26.75, -59.5)
  line L673 (26.75, -59.5) -> (26.75, -61)
  line L674 (26.75, -58.5) -> (35.25, -58.5)
  line L675 (35.25, -58.5) -> (35.25, -57)
  line L676 (35.25, -57) -> (26.75, -57)
  line L677 (26.75, -57) -> (26.75, -58.5)
  line L678 (26.75, -46) -> (35.25, -46)
  line L679 (35.25, -46) -> (35.25, -44.5)
  line L680 (35.25, -44.5) -> (26.75, -44.5)
  line L681 (26.75, -44.5) -> (26.75, -46)
  line L682 (26.75, -43.5) -> (35.25, -43.5)
  line L683 (35.25, -43.5) -> (35.25, -42)
  line L684 (35.25, -42) -> (26.75, -42)
  line L685 (26.75, -42) -> (26.75, -43.5)
  line L686 (26.75, -31) -> (35.25, -31)
  line L687 (35.25, -31) -> (35.25, -29.5)
  line L688 (35.25, -29.5) -> (26.75, -29.5)
  line L689 (26.75, -29.5) -> (26.75, -31)
  line L690 (26.75, -28.5) -> (35.25, -28.5)
  line L691 (35.25, -28.5) -> (35.25, -27)
  line L692 (35.25, -27) -> (26.75, -27)
  line L693 (26.75, -27) -> (26.75, -28.5)
  line L694 (26.75, -16) -> (35.25, -16)
  line L695 (35.25, -16) -> (35.25, -14.5)
  line L696 (35.25, -14.5) -> (26.75, -14.5)
  line L697 (26.75, -14.5) -> (26.75, -16)
  line L698 (26.75, -13.5) -> (35.25, -13.5)
  line L699 (35.25, -13.5) -> (35.25, -12)
  line L700 (35.25, -12) -> (26.75, -12)
  line L701 (26.75, -12) -> (26.75, -13.5)
  line L702 (26.75, -1) -> (35.25, -1)
  line L703 (35.25, -1) -> (35.25, 0.5)
  line L704 (35.25, 0.5) -> (26.75, 0.5)
  line L705 (26.75, 0.5) -> (26.75, -1)
  line L706 (26.75, 1.5) -> (35.25, 1.5)
  line L707 (35.25, 1.5) -> (35.25, 3)
  line L708 (35.25, 3) -> (26.75, 3)
  line L709 (26.75, 3) -> (26.75, 1.5)
  line L710 (26.75, 14) -> (35.25, 14)
  line L711 (35.25, 14) -> (35.25, 15.5)
  line L712 (35.25, 15.5) -> (26.75, 15.5)
  line L713 (26.75, 15.5) -> (26.75, 14)
  line L714 (26.75, 16.5) -> (35.25, 16.5)
  line L715 (35.25, 16.5) -> (35.25, 18)
  line L716 (35.25, 18) -> (26.75, 18)
  line L717 (26.75, 18) -> (26.75, 16.5)
  line L718 (26.75, 29) -> (35.25, 29)
  line L719 (35.25, 29) -> (35.25, 30.5)
  line L720 (35.25, 30.5) -> (26.75, 30.5)
  line L721 (26.75, 30.5) -> (26.75, 29)
  line L722 (26.75, 31.5) -> (35.25, 31.5)
  line L723 (35.25, 31.5) -> (35.25, 33)
  line L724 (35.25, 33) -> (26.75, 33)
  line L725 (26.75, 33) -> (26.75, 31.5)
  line L726 (26.75, 44) -> (35.25, 44)
  line L727 (35.25, 44) -> (35.25, 45.5)
  line L728 (35.25, 45.5) -> (26.75, 45.5)
  line L729 (26.75, 45.5) -> (26.75, 44)
  line L730 (26.75, 46.5) -> (35.25, 46.5)
  line L731 (35.25, 46.5) -> (35.25, 48)
  line L732 (35.25, 48) -> (26.75, 48)
  line L733 (26.75, 48) -> (26.75, 46.5)
  line L734 (26.75, 59) -> (35.25, 59)
  line L735 (35.25, 59) -> (35.25, 60.5)
  line L736 (35.25, 60.5) -> (26.75, 60.5)
  line L737 (26.75, 60.5) -> (26.75, 59)
  line L738 (26.75, 61.5) -> (35.25, 61.5)
  line L739 (35.25, 61.5) -> (35.25, 63)
  line L740 (35.25, 63) -> (26.75, 63)
  line L741 (26.75, 63) -> (26.75, 61.5)
  line L742 (26.75, 74) -> (35.25, 74)
  line L743 (35.25, 74) -> (35.25, 75.5)
  line L744 (35.25, 75.5) -> (26.75, 75.5)
  line L745 (26.75, 75.5) -> (26.75, 74)
  line L746 (26.75, 76.5) -> (35.25, 76.5)
  line L747 (35.25, 76.5) -> (35.25, 78)
  line L748 (35.25, 78) -> (26.75, 78)
  line L749 (26.75, 78) -> (26.75, 76.5)
  line L750 (26.75, 89) -> (35.25, 89)
  line L751 (35.25, 89) -> (35.25, 90.5)
  line L752 (35.25, 90.5) -> (26.75, 90.5)
  line L753 (26.75, 90.5) -> (26.75, 89)
  line L754 (26.75, 91.5) -> (35.25, 91.5)
  line L755 (35.25, 91.5) -> (35.25, 93)
  line L756 (35.25, 93) -> (26.75, 93)
  line L757 (26.75, 93) -> (26.75, 91.5)
  line L758 (26.75, 104) -> (35.25, 104)
  line L759 (35.25, 104) -> (35.25, 105.5)
  line L760 (35.25, 105.5) -> (26.75, 105.5)
  line L761 (26.75, 105.5) -> (26.75, 104)
  line L762 (26.75, 106.5) -> (35.25, 106.5)
  line L763 (35.25, 106.5) -> (35.25, 108)
  line L764 (35.25, 108) -> (26.75, 108)
  line L765 (26.75, 108) -> (26.75, 106.5)
  line L766 (26.75, 119) -> (35.25, 119)
  line L767 (35.25, 119) -> (35.25, 120.5)
  line L768 (35.25, 120.5) -> (26.75, 120.5)
  line L769 (26.75, 120.5) -> (26.75, 119)
  line L770 (41.75, -118.5) -> (50.25, -118.5)
  line L771 (50.25, -118.5) -> (50.25, -117)
  line L772 (50.25, -117) -> (41.75, -117)
  line L773 (41.75, -117) -> (41.75, -118.5)
  line L774 (41.75, -106) -> (50.25, -106)
  line L775 (50.25, -106) -> (50.25, -104.5)
  line L776 (50.25, -104.5) -> (41.75, -104.5)
  line L777 (41.75, -104.5) -> (41.75, -106)
  line L778 (41.75, -103.5) -> (50.25, -103.5)
  line L779 (50.25, -103.5) -> (50.25, -102)
  line L780 (50.25, -102) -> (41.75, -102)
  line L781 (41.75, -102) -> (41.75, -103.5)
  line L782 (41.75, -91) -> (50.25, -91)
  line L783 (50.25, -91) -> (50.25, -89.5)
  line L784 (50.25, -89.5) -> (41.75, -89.5)
  line L785 (41.75, -89.5) -> (41.75, -91)
  line L786 (41.75, -88.5) -> (50.25, -88.5)
  line L787 (50.25, -88.5) -> (50.25, -87)
  line L788 (50.25, -87) -> (41.75, -87)
  line L789 (41.75, -87) -> (41.75, -88.5)
  line L790 (41.75, -76) -> (50.25, -76)
  line L791 (50.25, -76) -> (50.25, -74.5)
  line L792 (50.25, -74.5) -> (41.75, -74.5)
  line L793 (41.75, -74.5) -> (41.75, -76)
  line L794 (41.75, -73.5) -> (50.25, -73.5)
  line L795 (50.25, -73.5) -> (50.25, -72)
  line L796 (50.25, -72) -> (41.75, -72)
  line L797 (41.75, -72) -> (41.75, -73.5)
  line L798 (41.75, -61) -> (50.25, -61)
  line L799 (50.25, -61) -> (50.25, -59.5)
  line L800 (50.25, -59.5) -> (41.75, -59.5)
  line L801 (41.75, -59.5) -> (41.75, -61)
  line L802 (41.75, -58.5) -> (50.25, -58.5)
  line L803 (50.25, -58.5) -> (50.25, -57)
  line L804 (50.25, -57) -> (41.75, -57)
  line L805 (41.75, -57) -> (41.75, -58.5)
  line L806 (41.75, -46) -> (50.25, -46)
  line L807 (50.25, -46) -> (50.25, -44.5)
  line L808 (50.25, -44.5) -> (41.75, -44.5)
  line L809 (41.75, -44.5) -> (41.75, -46)
  line L810 (41.75, -43.5) -> (50.25, -43.5)
  line L811 (50.25, -43.5) -> (50.25, -42)
  line L812 (50.25, -42) -> (41.75, -42)
  line L813 (41.75, -42) -> (41.75, -43.5)
  line L814 (41.75, -31) -> (50.25, -31)
  line L815 (50.25, -31) -> (50.25, -29.5)
  line L816 (50.25, -29.5) -> (41.75, -29.5)
  line L817 (41.75, -29.5) -> (41.75, -31)
  line L818 (41.75, -28.5) -> (50.25, -28.5)
  line L819 (50.25, -28.5) -> (50.25, -27)
  line L820 (50.25, -27) -> (41.75, -27)
  line L821 (41.75, -27) -> (41.75, -28.5)
  line L822 (41.75, -16) -> (50.25, -16)
  line L823 (50.25, -16) -> (50.25, -14.5)
  line L824 (50.25, -14.5) -> (41.75, -14.5)
  line L825 (41.75, -14.5) -> (41.75, -16)
  line L826 (41.75, -13.5) -> (50.25, -13.5)
  line L827 (50.25, -13.5) -> (50.25, -12)
  line L828 (50.25, -12) -> (41.75, -12)
  line L829 (41.75, -12) -> (41.75, -13.5)
  line L830 (41.75, -1) -> (50.25, -1)
  line L831 (50.25, -1) -> (50.25, 0.5)
  line L832 (50.25, 0.5) -> (41.75, 0.5)
  line L833 (41.75, 0.5) -> (41.75, -1)
  line L834 (41.75, 1.5) -> (50.25, 1.5)
  line L835 (50.25, 1.5) -> (50.25, 3)
  line L836 (50.25, 3) -> (41.75, 3)
  line L837 (41.75, 3) -> (41.75, 1.5)
  line L838 (41.75, 14) -> (50.25, 14)
  line L839 (50.25, 14) -> (50.25, 15.5)
  line L840 (50.25, 15.5) -> (41.75, 15.5)
  line L841 (41.75, 15.5) -> (41.75, 14)
  line L842 (41.75, 16.5) -> (50.25, 16.5)
  line L843 (50.25, 16.5) -> (50.25, 18)
  line L844 (50.25, 18) -> (41.75, 18)
  line L845 (41.75, 18) -> (41.75, 16.5)
  line L846 (41.75, 29) -> (50.25, 29)
  line L847 (50.25, 29) -> (50.25, 30.5)
  line L848 (50.25, 30.5) -> (41.75, 30.5)
  line L849 (41.75, 30.5) -> (41.75, 29)
  line L850 (41.75, 31.5) -> (50.25, 31.5)
  line L851 (50.25, 31.5) -> (50.25, 33)
  line L852 (50.25, 33) -> (41.75, 33)
  line L853 (41.75, 33) -> (41.75, 31.5)
  line L854 (41.75, 44) -> (50.25, 44)
  line L855 (50.25, 44) -> (50.25, 45.5)
  line L856 (50.25, 45.5) -> (41.75, 45.5)
  line L857 (41.75, 45.5) -> (41.75, 44)
  line L858 (41.75, 46.5) -> (50.25, 46.5)
  line L859 (50.25, 46.5) -> (50.25, 48)
  line L860 (50.25, 48) -> (41.75, 48)
  line L861 (41.75, 48) -> (41.75, 46.5)
  line L862 (41.75, 59) -> (50.25, 59)
  line L863 (50.25, 59) -> (50.25, 60.5)
  line L864 (50.25, 60.5) -> (41.75, 60.5)
  line L865 (41.75, 60.5) -> (41.75, 59)
  line L866 (41.75, 61.5) -> (50.25, 61.5)
  line L867 (50.25, 61.5) -> (50.25, 63)
  line L868 (50.25, 63) -> (41.75, 63)
  line L869 (41.75, 63) -> (41.75, 61.5)
  line L870 (41.75, 74) -> (50.25, 74)
  line L871 (50.25, 74) -> (50.25, 75.5)
  line L872 (50.25, 75.5) -> (41.75, 75.5)
  line L873 (41.75, 75.5) -> (41.75, 74)
  line L874 (41.75, 76.5) -> (50.25, 76.5)
  line L875 (50.25, 76.5) -> (50.25, 78)
  line L876 (50.25, 78) -> (41.75, 78)
  line L877 (41.75, 78) -> (41.75, 76.5)
  line L878 (41.75, 89) -> (50.25, 89)
  line L879 (50.25, 89) -> (50.25, 90.5)
  line L880 (50.25, 90.5) -> (41.75, 90.5)
  line L881 (41.75, 90.5) -> (41.75, 89)
  line L882 (41.75, 91.5) -> (50.25, 91.5)
  line L883 (50.25, 91.5) -> (50.25, 93)
  line L884 (50.25, 93) -> (41.75, 93)
  line L885 (41.75, 93) -> (41.75, 91.5)
  line L886 (41.75, 104) -> (50.25, 104)
  line L887 (50.25, 104) -> (50.25, 105.5)
  line L888 (50.25, 105.5) -> (41.75, 105.5)
  line L889 (41.75, 105.5) -> (41.75, 104)
  line L890 (41.75, 106.5) -> (50.25, 106.5)
  line L891 (50.25, 106.5) -> (50.25, 108)
  line L892 (50.25, 108) -> (41.75, 108)
  line L893 (41.75, 108) -> (41.75, 106.5)
  line L894 (41.75, 119) -> (50.25, 119)
  line L895 (50.25, 119) -> (50.25, 120.5)
  line L896 (50.25, 120.5) -> (41.75, 120.5)
  line L897 (41.75, 120.5) -> (41.75, 119)
  line L898 (11.75, -68.5) -> (20.25, -68.5)
  line L899 (20.25, -68.5) -> (20.25, -67)
  line L900 (20.25, -67) -> (11.75, -67)
  line L901 (11.75, -67) -> (11.75, -68.5)
  line L902 (60.5, -129.5) -> (60.5, 131.5) projected
  line L903 (11.75, -64.5) -> (20.25, -64.5)
  line L904 (20.25, -64.5) -> (20.25, -66)
  line L905 (20.25, -66) -> (11.75, -66)
  line L906 (11.75, -66) -> (11.75, -64.5)
  line L907 (11.75, -53.5) -> (20.25, -53.5)
  line L908 (20.25, -53.5) -> (20.25, -52)
  line L909 (20.25, -52) -> (11.75, -52)
  line L910 (11.75, -52) -> (11.75, -53.5)
  line L911 (11.75, -51) -> (20.25, -51)
  line L912 (20.25, -51) -> (20.25, -49.5)
  line L913 (20.25, -49.5) -> (11.75, -49.5)
  line L914 (11.75, -49.5) -> (11.75, -51)
  line L915 (11.75, -8.5) -> (20.25, -8.5)
  line L916 (20.25, -8.5) -> (20.25, -7)
  line L917 (20.25, -7) -> (11.75, -7)
  line L918 (11.75, -7) -> (11.75, -8.5)
  line L919 (11.75, -6) -> (20.25, -6)
  line L920 (20.25, -6) -> (20.25, -4.5)
  line L921 (20.25, -4.5) -> (11.75, -4.5)
  line L922 (11.75, -4.5) -> (11.75, -6)
  line L923 (11.75, 36.5) -> (20.25, 36.5)
  line L924 (20.25, 36.5) -> (20.25, 38)
  line L925 (20.25, 38) -> (11.75, 38)
  line L926 (11.75, 38) -> (11.75, 36.5)
  line L927 (11.75, 39) -> (20.25, 39)
  line L928 (20.25, 39) -> (20.25, 40.5)
  line L929 (20.25, 40.5) -> (11.75, 40.5)
  line L930 (11.75, 40.5) -> (11.75, 39)
  line L931 (11.75, 51.5) -> (20.25, 51.5)
  line L932 (20.25, 51.5) -> (20.25, 53)
  line L933 (20.25, 53) -> (11.75, 53)
  line L934 (11.75, 53) -> (11.75, 51.5)
  line L935 (11.75, 54) -> (20.25, 54)
  line L936 (20.25, 54) -> (20.25, 55.5)
  line L937 (20.25, 55.5) -> (11.75, 55.5)
  line L938 (11.75, 55.5) -> (11.75, 54)
  point P0 (0, 0)
  dimension "d93" = 8.5
  dimension "d94" = 1.5
  dimension "d95" = 1.5
  dimension "d96" = 11
  dimension "d97" = 13.75
  dimension "d98" = 11
  dimension "d101" = 15
  dimension "d104" = 15
  dimension "d111" = 8.5
  dimension "d112" = 1.5
  dimension "d113" = 18.5
  dimension "d115" = 8.5
  dimension "d116" = 1.5
  dimension "d117" = 1.5
  dimension "d118" = 1
  dimension "d119" = 11
  dimension "d120" = 8.5
  dimension "d121" = 8.5
  dimension "d122" = 8.5
  dimension "d123" = 1.5
  dimension "d124" = 18.5
  dimension "d125" = 8.5
  dimension "d126" = 8.5
  dimension "d127" = 1.5
  dimension "d128" = 1.5
  dimension "d129" = 18.5
  dimension "d130" = 18.5
  dimension "d131" = 8.5
  dimension "d132" = 1.5
  dimension "d133" = 1.5
  dimension "d134" = 1.5
  dimension "d135" = 1.5
  dimension "d136" = 18.5
  dimension "d137" = 1
  dimension "d138" = 11
  dimension "d139" = 18.5
  dimension "d140" = 8.5
  constraints: 1872 end point, 232 point on line, 24 parallel, 13 horizontal, 12 perpendicular, 1 vertical, 1776 other
  measures "d93" distance of L5.end L6.end
  measures "d94" distance of L2.end L0.start
  measures "d95" distance of L6.end L4.start
  measures "d96" distance between parallel lines of L2 L4
  measures "d97" distance between parallel lines of L8 L3
  measures "d98" distance between parallel lines of L9 L0
  measures "d101" distance of L0.start L10.start
  measures "d104" distance of L0.start L130.start
  measures "d111" distance of L899.end L900.end
  measures "d112" distance of L900.end L898.start
  measures "d113" distance between parallel lines of L532 L898
  measures "d115" distance between parallel lines of L541 L899
  measures "d116" distance of L907.end L908.end
  measures "d117" distance of L903.end L904.end
  measures "d118" distance between parallel lines of L900 L905
  measures "d119" distance between parallel lines of L907 L903
  measures "d120" distance between parallel lines of L547 L910
  measures "d121" distance between parallel lines of L545 L904
  measures "d122" distance of L912.end L913.end
  measures "d123" distance of L913.end L911.start
  measures "d124" distance between parallel lines of L913 L558
  measures "d125" distance between parallel lines of L553 L912
  measures "d126" distance of L915.start L915.end
  measures "d127" distance of L915.end L916.end
  measures "d128" distance of L919.end L920.end
  measures "d129" distance between parallel lines of L564 L915
  measures "d130" distance between parallel lines of L921 L582
  measures "d131" distance between parallel lines of L571 L918
  measures "d132" distance of L923.end L924.end
  measures "d133" distance of L927.end L928.end
  measures "d134" distance of L933.end L931.start
  measures "d135" distance of L937.end L935.start
  measures "d136" distance between parallel lines of L588 L923
  measures "d137" distance between parallel lines of L925 L927
  measures "d138" distance between parallel lines of L929 L931
  measures "d139" distance between parallel lines of L937 L614
  measures "d140" distance between parallel lines of L595 L926
body "Solid1"
